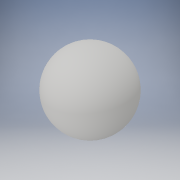
# Autodesk Inventor part: bearing6mm
Saved by Autodesk Inventor 2018 (Build 220112000, 112)
## iProperties
Created: 2020-03-27
Part Number: bearing6mm
Material: Generic
Document SubType Name: Modeling
Designer: natha
Density: 1 g/cm^3
Appearance: Default
Author: natha
Autodesk Inventor part; units mm, degrees
ref_plane "YZ Plane" through (0, 0, 0) normal (1, 0, 0) x (0, 1, 0)
ref_plane "XZ Plane" through (0, 0, 0) normal (0, 1, 0) x (-1, 0, 0)
ref_plane "XY Plane" through (0, 0, 0) normal (0, 0, 1) x (1, 0, 0)
sketch "Sketch1" plane through (0, 0, 0) normal (0, 1, 0) x (-1, 0, 0)
  arc A0 (3, 0) -> (0, 3) centre (0, 0) ccw
  arc A1 (0, 3) -> (-3, 0) centre (0, 0) ccw
  line L0 (3, 0) -> (-3, 0)
  dimension "d1" = 3
  constraints: 4 point on circle, 2 centre point, 2 coincident, 2 end point, 1 horizontal
  measures "d1" radius of A0
revolve "Revolution1" add sketch "Sketch1" angle 360 about axis through (-3, 0, 0) along (-1, 0, 0)
body "Solid1"
